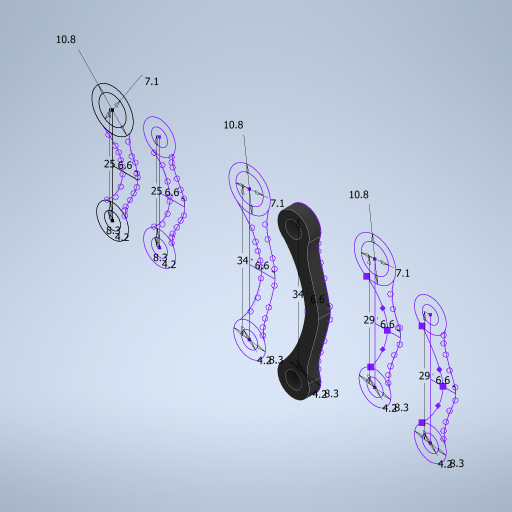
# Autodesk Inventor part: Leg_Front_V5_b
Saved by Autodesk Inventor 2023.1 (Build 271208000, 208)
## iProperties
Created: 2022-10-11
Part Number: Leg_Front_V5_b
Material: Rubber, Silicone
Document SubType Name: Modeling
Designer: Windows10
Density: 1.25 g/cm^3
Appearance: Rubber - Black
Author: Windows10
Autodesk Inventor part; units mm, degrees
ref_plane "YZ Plane" through (0, 0, 0) normal (1, 0, 0) x (0, 1, 0)
ref_plane "XZ Plane" through (0, 0, 0) normal (0, 1, 0) x (-1, 0, 0)
ref_plane "XY Plane" through (0, 0, 0) normal (0, 0, 1) x (1, 0, 0)
sketch "Sketch1" plane through (0, 0, 0) normal (0, 0, 1) x (1, 0, 0)
  circle A0 centre (0, 0) radius 5.4
  line L0 (0, 0) -> (0, -25)
  circle A1 centre (0, -25) radius 4.15
  circle A2 centre (0, -25) radius 2.1
  line L1 (0, -12.5) -> (6.6, -12.5)
  circle A3 centre (0, 0) radius 3.55
  line L2 (4.5636, -2.8868) -> (4.15, -5.0505) construction
  line L3 (4.15, -5.0505) -> (5.1368, -7.8346) construction
  line L4 (5.1368, -7.8346) -> (6.0268, -8.8456) construction
  line L5 (6.0268, -8.8456) -> (6.4445, -11.0297) construction
  line L6 (6.4445, -11.0297) -> (6.6598, -11.8582) construction
  line L7 (6.6598, -11.8582) -> (6.6, -12.5) construction
  spline S0 degree 4 poles (4.5636, -2.8868) (4.15, -5.0505) (5.1368, -7.8346) (6.0268, -8.8456) (6.4445, -11.0297) (6.6598, -11.8582) (6.6, -12.5) knots 1 1 1 1 1 2 3 4 4 4 4 4
  line L8 (-2.6712, -4.6931) -> (-0.9445, -6.0036) construction
  line L9 (-0.9445, -6.0036) -> (0.8697, -7.604) construction
  line L10 (0.8697, -7.604) -> (1.7388, -8.6572) construction
  line L11 (1.7388, -8.6572) -> (2.2595, -10.1019) construction
  line L12 (2.2595, -10.1019) -> (2.7672, -11.4262) construction
  line L13 (2.7672, -11.4262) -> (2.7672, -12.5) construction
  spline S1 degree 4 poles (-2.6712, -4.6931) (-0.9445, -6.0036) (0.8697, -7.604) (1.7388, -8.6572) (2.2595, -10.1019) (2.7672, -11.4262) (2.7672, -12.5) knots 1 1 1 1 1 2 3 4 4 4 4 4
  line L14 (2.7672, -12.5) -> (2.7672, -13.0618) construction
  line L15 (2.7672, -13.0618) -> (2.2595, -16.1544) construction
  line L16 (2.2595, -16.1544) -> (0.8697, -19.1754) construction
  line L17 (0.8697, -19.1754) -> (-1.323, -20.85) construction
  line L18 (-1.323, -20.85) -> (-2.1, -21.4205) construction
  spline S2 degree 4 poles (2.7672, -12.5) (2.7672, -13.0618) (2.2595, -16.1544) (0.8697, -19.1754) (-1.323, -20.85) (-2.1, -21.4205) knots 1 1 1 1 1 2 3 3 3 3 3
  line L19 (6.6, -12.5) -> (6.4445, -14.1704) construction
  line L20 (6.4445, -14.1704) -> (5.6131, -15.9877) construction
  line L21 (5.6131, -15.9877) -> (4.6434, -17.9759) construction
  line L22 (4.6434, -17.9759) -> (3.55, -20.0127) construction
  line L23 (3.55, -20.0127) -> (3.3, -20.9586) construction
  line L24 (3.3, -20.9586) -> (3.3, -22.207) construction
  line L25 (3.3, -22.207) -> (3.7922, -23.3143) construction
  spline S3 degree 4 poles (6.6, -12.5) (6.4445, -14.1704) (5.6131, -15.9877) (4.6434, -17.9759) (3.55, -20.0127) (3.3, -20.9586) (3.3, -22.207) (3.7922, -23.3143) knots 1 1 1 1 1 2 3 4 5 5 5 5 5
  circle A4 centre (35.7502, 0) radius 5.4
  circle A5 centre (35.7502, 0) radius 3.55
  line L26 (12.2485, 0) -> (12.2485, -25)
  circle A6 centre (12.2485, -25) radius 4.15
  circle A7 centre (12.2485, -25) radius 2.1
  line L27 (12.2485, -12.5) -> (18.8485, -12.5)
  line L28 (15.0157, -12.5) -> (15.0157, -13.0618) construction
  line L29 (15.0157, -13.0618) -> (14.5079, -16.1544) construction
  line L30 (14.5079, -16.1544) -> (13.1182, -19.1754) construction
  line L31 (13.1182, -19.1754) -> (10.9255, -20.85) construction
  line L32 (10.9255, -20.85) -> (10.1485, -21.4205) construction
  spline S4 degree 4 poles (15.0157, -12.5) (15.0157, -13.0618) (14.5079, -16.1544) (13.1182, -19.1754) (10.9255, -20.85) (10.1485, -21.4205) knots 1 1 1 1 1 2 3 3 3 3 3
  line L33 (18.8485, -12.5) -> (18.7327, -14.3682) construction
  line L34 (18.7327, -14.3682) -> (17.8616, -15.9877) construction
  line L35 (17.8616, -15.9877) -> (16.8918, -17.9759) construction
  line L36 (16.8918, -17.9759) -> (15.7985, -20.0127) construction
  line L37 (15.7985, -20.0127) -> (15.5485, -20.9586) construction
  line L38 (15.5485, -20.9586) -> (15.5485, -22.207) construction
  line L39 (15.5485, -22.207) -> (16.0407, -23.3143) construction
  spline S5 degree 4 poles (18.8485, -12.5) (18.7327, -14.3682) (17.8616, -15.9877) (16.8918, -17.9759) (15.7985, -20.0127) (15.5485, -20.9586) (15.5485, -22.207) (16.0407, -23.3143) knots 1 1 1 1 1 2 3 4 5 5 5 5 5
  line L40 (18.8485, -12.5) -> (18.7327, -10.6318) construction
  spline S6 degree 4 poles (18.8485, -12.5) (18.7327, -10.6318) (17.8616, -9.0123) (16.8918, -7.0241) (15.7985, -4.9873) (15.5485, -4.0414) (15.5485, -2.793) (16.0407, -1.6857) knots 1 1 1 1 1 2 3 4 5 5 5 5 5
  line L41 (18.7327, -10.6318) -> (17.8616, -9.0123) construction
  line L42 (17.8616, -9.0123) -> (16.8918, -7.0241) construction
  line L43 (16.8918, -7.0241) -> (15.7985, -4.9873) construction
  line L44 (15.7985, -4.9873) -> (15.5485, -4.0414) construction
  line L45 (15.5485, -4.0414) -> (15.5485, -2.793) construction
  line L46 (15.5485, -2.793) -> (16.0407, -1.6857) construction
  line L47 (14.5079, -8.8456) -> (13.1182, -5.8246) construction
  spline S7 degree 4 poles (15.0157, -12.5) (15.0157, -11.9382) (14.5079, -8.8456) (13.1182, -5.8246) (10.9255, -4.15) (10.1485, -3.5795) knots 1 1 1 1 1 2 3 3 3 3 3
  line L48 (15.0157, -12.5) -> (15.0157, -11.9382) construction
  line L49 (15.0157, -11.9382) -> (14.5079, -8.8456) construction
  line L50 (13.1182, -5.8246) -> (10.9255, -4.15) construction
  line L51 (10.9255, -4.15) -> (10.1485, -3.5795) construction
  circle A8 centre (12.2485, 0) radius 2.1
  circle A9 centre (12.2485, 0) radius 4.15
  line L52 (35.7502, 0) -> (35.7502, -34)
  circle A10 centre (35.7502, -34) radius 2.1
  circle A11 centre (35.7502, -34) radius 4.15
  line L53 (35.7502, -17) -> (42.3502, -17)
  line L54 (40.7252, -2.1) -> (39.9002, -5.8246) construction
  line L55 (39.9002, -5.8246) -> (40.5798, -8.8456) construction
  line L56 (40.5798, -8.8456) -> (41.8697, -12.5) construction
  line L57 (41.8697, -12.5) -> (42.3502, -14.707) construction
  line L58 (42.3502, -14.707) -> (42.3502, -17) construction
  spline S8 degree 4 poles (40.7252, -2.1) (39.9002, -5.8246) (40.5798, -8.8456) (41.8697, -12.5) (42.3502, -14.707) (42.3502, -17) knots 1 1 1 1 1 2 3 3 3 3 3
  line L59 (32.2762, -4.1341) -> (36.4644, -8.3401) construction
  line L60 (36.4644, -8.3401) -> (37.406, -11.0297) construction
  line L61 (37.406, -11.0297) -> (38.0185, -12.7794) construction
  line L62 (38.0185, -12.7794) -> (38.6784, -14.6643) construction
  line L63 (38.6784, -14.6643) -> (38.8308, -15.9862) construction
  line L64 (38.8308, -15.9862) -> (38.8308, -17) construction
  spline S9 degree 4 poles (32.2762, -4.1341) (36.4644, -8.3401) (37.406, -11.0297) (38.0185, -12.7794) (38.6784, -14.6643) (38.8308, -15.9862) (38.8308, -17) knots 1 1 1 1 1 2 3 4 4 4 4 4
  line L65 (38.8308, -17) -> (38.8308, -18.5598) construction
  line L66 (38.8308, -18.5598) -> (38.0185, -23.3143) construction
  line L67 (38.0185, -23.3143) -> (36.1571, -27.3727) construction
  line L68 (36.1571, -27.3727) -> (33.2415, -30.6942) construction
  spline S10 degree 4 poles (38.8308, -17) (38.8308, -18.5598) (38.0185, -23.3143) (36.1571, -27.3727) (33.2415, -30.6942) knots 1 1 1 1 1 2 2 2 2 2
  line L69 (42.3502, -17) -> (42.3502, -18.4687) construction
  line L70 (42.3502, -18.4687) -> (40.8654, -24.0864) construction
  line L71 (40.8654, -24.0864) -> (39.9002, -27.1) construction
  line L72 (39.9002, -27.1) -> (39.3002, -29.3894) construction
  line L73 (39.3002, -29.3894) -> (39.3002, -31.2196) construction
  line L74 (39.3002, -31.2196) -> (39.758, -32.9229) construction
  spline S11 degree 4 poles (42.3502, -17) (42.3502, -18.4687) (40.8654, -24.0864) (39.9002, -27.1) (39.3002, -29.3894) (39.3002, -31.2196) (39.758, -32.9229) knots 1 1 1 1 1 2 3 4 4 4 4 4
  line L75 (50.1975, -0.3995) -> (50.1975, -34.3995)
  circle A12 centre (50.1975, -34.3995) radius 2.1
  circle A13 centre (50.1975, -34.3995) radius 4.15
  line L76 (50.1975, -17.3995) -> (56.7975, -17.3995)
  line L77 (53.2781, -17.3995) -> (53.2781, -18.9593) construction
  line L78 (53.2781, -18.9593) -> (52.4658, -23.7138) construction
  line L79 (52.4658, -23.7138) -> (50.6044, -27.7721) construction
  line L80 (50.6044, -27.7721) -> (47.6887, -31.0936) construction
  spline S12 degree 4 poles (53.2781, -17.3995) (53.2781, -18.9593) (52.4658, -23.7138) (50.6044, -27.7721) (47.6887, -31.0936) knots 1 1 1 1 1 2 2 2 2 2
  line L81 (56.7975, -17.3995) -> (56.7975, -18.8682) construction
  line L82 (56.7975, -18.8682) -> (55.3127, -24.4859) construction
  line L83 (55.3127, -24.4859) -> (54.3475, -27.4995) construction
  line L84 (54.3475, -27.4995) -> (53.7475, -29.7889) construction
  line L85 (53.7475, -29.7889) -> (53.7475, -31.619) construction
  line L86 (53.7475, -31.619) -> (54.2053, -33.3224) construction
  spline S13 degree 4 poles (56.7975, -17.3995) (56.7975, -18.8682) (55.3127, -24.4859) (54.3475, -27.4995) (53.7475, -29.7889) (53.7475, -31.619) (54.2053, -33.3224) knots 1 1 1 1 1 2 3 4 4 4 4 4
  line L87 (56.7975, -17.3995) -> (56.7975, -15.9308) construction
  spline S14 degree 4 poles (56.7975, -17.3995) (56.7975, -15.9308) (55.3127, -10.3131) (54.3475, -7.2995) (53.7475, -5.0101) (53.7475, -3.1799) (54.2053, -1.4766) knots 1 1 1 1 1 2 3 4 4 4 4 4
  line L88 (56.7975, -15.9308) -> (55.3127, -10.3131) construction
  line L89 (55.3127, -10.3131) -> (54.3475, -7.2995) construction
  line L90 (54.3475, -7.2995) -> (53.7475, -5.0101) construction
  line L91 (53.7475, -5.0101) -> (53.7475, -3.1799) construction
  line L92 (53.7475, -3.1799) -> (54.2053, -1.4766) construction
  line L93 (53.2781, -17.3995) -> (53.2781, -15.8397) construction
  spline S15 degree 4 poles (53.2781, -17.3995) (53.2781, -15.8397) (52.4658, -11.0852) (50.6044, -7.0268) (47.6887, -3.7053) knots 1 1 1 1 1 2 2 2 2 2
  line L94 (53.2781, -15.8397) -> (52.4658, -11.0852) construction
  line L95 (52.4658, -11.0852) -> (50.6044, -7.0268) construction
  line L96 (50.6044, -7.0268) -> (47.6887, -3.7053) construction
  circle A14 centre (50.1975, -0.3995) radius 2.1
  circle A15 centre (50.1975, -0.3995) radius 4.15
  circle A16 centre (68.4548, 0.5836) radius 5.4
  circle A17 centre (68.4548, 0.5836) radius 3.55
  line L97 (68.4548, 0.5836) -> (68.4548, -28.4164)
  circle A18 centre (68.4548, -28.4164) radius 2.1
  circle A19 centre (68.4548, -28.4164) radius 4.15
  line L98 (68.4548, -13.9164) -> (75.0548, -13.9164)
  line L99 (73.4297, -1.5164) -> (72.6048, -5.241) construction
  line L100 (72.6048, -5.241) -> (73.2844, -8.262) construction
  line L101 (73.2844, -8.262) -> (74.5743, -11.9164) construction
  line L102 (74.5743, -11.9164) -> (75.0548, -11.6234) construction
  line L103 (75.0548, -11.6234) -> (75.0548, -13.9164) construction
  spline S16 degree 4 poles (73.4297, -1.5164) (72.6048, -5.241) (73.2844, -8.262) (74.5743, -11.9164) (75.0548, -11.6234) (75.0548, -13.9164) knots 1 1 1 1 1 2 3 3 3 3 3
  line L104 (75.0548, -13.9164) -> (75.0548, -15.3851) construction
  line L105 (75.0548, -15.3851) -> (73.57, -18.5028) construction
  line L106 (73.57, -18.5028) -> (72.6048, -21.5164) construction
  line L107 (72.6048, -21.5164) -> (72.0048, -23.8058) construction
  line L108 (72.0048, -23.8058) -> (72.0048, -25.636) construction
  line L109 (72.0048, -25.636) -> (72.4626, -27.3393) construction
  spline S17 degree 4 poles (75.0548, -13.9164) (75.0548, -15.3851) (73.57, -18.5028) (72.6048, -21.5164) (72.0048, -23.8058) (72.0048, -25.636) (72.4626, -27.3393) knots 1 1 1 1 1 2 3 4 4 4 4 4
  line L110 (89.5021, -19.3159) -> (89.5021, -20.7846) construction
  spline S18 degree 4 poles (89.5021, -19.3159) (89.5021, -20.7846) (88.0172, -23.9023) (87.0521, -26.9159) (86.4521, -29.2053) (86.4521, -31.0355) (86.9099, -32.7388) knots 1 1 1 1 1 2 3 4 4 4 4 4
  line L111 (89.5021, -20.7846) -> (88.0172, -23.9023) construction
  line L112 (88.0172, -23.9023) -> (87.0521, -26.9159) construction
  line L113 (87.0521, -26.9159) -> (86.4521, -29.2053) construction
  line L114 (86.4521, -29.2053) -> (86.4521, -31.0355) construction
  line L115 (86.4521, -31.0355) -> (86.9099, -32.7388) construction
  line L116 (82.9021, -19.3159) -> (89.5021, -19.3159)
  line L117 (82.9021, -4.8159) -> (82.9021, -33.8159)
  circle A20 centre (82.9021, -33.8159) radius 2.1
  circle A21 centre (82.9021, -33.8159) radius 4.15
  spline S19 degree 4 poles (89.5021, -19.3159) (89.5021, -17.8472) (88.0172, -14.7295) (87.0521, -11.7159) (86.4521, -9.4265) (86.4521, -7.5964) (86.9099, -5.893) knots 1 1 1 1 1 2 3 4 4 4 4 4
  line L118 (89.5021, -19.3159) -> (89.5021, -17.8472) construction
  line L119 (89.5021, -17.8472) -> (88.0172, -14.7295) construction
  line L120 (88.0172, -14.7295) -> (87.0521, -11.7159) construction
  line L121 (87.0521, -11.7159) -> (86.4521, -9.4265) construction
  line L122 (86.4521, -9.4265) -> (86.4521, -7.5964) construction
  line L123 (86.4521, -7.5964) -> (86.9099, -5.893) construction
  circle A22 centre (82.9021, -4.8159) radius 4.15
  circle A23 centre (82.9021, -4.8159) radius 2.1
  spline S20 degree 2 poles (80.8021, -8.3954) (86.1209, -15.5699) (86.2021, -19.3159) knots 0 0 0 1 1 1
  spline S21 degree 2 poles (80.8021, -30.2365) (86.0382, -24.7359) (86.2021, -19.3159) knots 0 0 0 1 1 1
  spline S22 degree 2 poles (67.394, -24.4043) (71.2801, -19.0052) (71.7548, -13.9164) knots 0 0 0 1 1 1
  spline S23 degree 2 poles (66.3548, -4.3914) (71.6414, -8.8733) (71.7548, -13.9164) knots 0 0 0 1 1 1
  point P0 (53.2056, -19.8995)
  point P1 (85.3498, -15.891)
  point P2 (85.0021, -24.2664)
  point P3 (70.5719, -18.7259)
  point P4 (70.5719, -9.4265)
  dimension "d0" = 10.8
  dimension "d1" = 25
  dimension "d2" = 8.3
  dimension "d3" = 4.2
  dimension "d4" = 6.6
  dimension "d5" = 7.1
  dimension "d8" = 10.8
  dimension "d9" = 7.1
  dimension "d11" = 25
  dimension "d12" = 8.3
  dimension "d13" = 4.2
  dimension "d14" = 6.6
  dimension "d18" = 34
  dimension "d19" = 4.2
  dimension "d20" = 8.3
  dimension "d21" = 6.6
  dimension "d24" = 34
  dimension "d25" = 4.2
  dimension "d26" = 8.3
  dimension "d27" = 6.6
  dimension "d32" = 10.8
  dimension "d33" = 7.1
  dimension "d34" = 29
  dimension "d35" = 4.2
  dimension "d36" = 8.3
  dimension "d37" = 6.6
  dimension "d38" = 29
  dimension "d39" = 4.2
  dimension "d40" = 8.3
  dimension "d41" = 6.6
  constraints: 34 symmetric about line, 24 centre point, 24 end point, 24 point on circle, 22 vertical, 19 coincident, 8 midpoint, 6 horizontal, 6 tangent, 4 point on line, 2 perpendicular, 1 collinear, 78 other
  measures "d0" diameter of A0
  measures "d1" distance of L0.start L0.end
  measures "d2" diameter of A1
  measures "d3" diameter of A2
  measures "d4" distance of L1.start L1.end
  measures "d5" diameter of A3
  measures "d8" diameter of A4
  measures "d9" diameter of A5
  measures "d11" distance of L26.start L26.end
  measures "d12" diameter of A6
  measures "d13" diameter of A7
  measures "d14" distance of L27.start L33.start
  measures "d18" distance of L52.start L52.end
  measures "d19" diameter of A10
  measures "d20" diameter of A11
  measures "d21" distance of L53.start L53.end
  measures "d24" distance of L75.start L75.end
  measures "d25" diameter of A12
  measures "d26" diameter of A13
  measures "d27" distance of L76.start L81.start
  measures "d32" diameter of A16
  measures "d33" diameter of A17
  measures "d34" distance of L97.start L97.end
  measures "d35" diameter of A18
  measures "d36" diameter of A19
  measures "d37" distance of L98.start L98.end
  measures "d38" distance of L117.start L117.end
  measures "d39" diameter of A20
  measures "d40" diameter of A21
  measures "d41" distance of L116.start L110.start
extrude "Extrusion1" add sketch "Sketch1" along normal blind 3 contours A0 | A0 L0 S1 | S0 L1 S1 L0 A0 | S3 A1 L0 S2 L1 | A1 | L0 A1 S2
extrude "Extrusion2" add sketch "Sketch1" along normal blind 3 separate body contours A9 | A9 S6 L27 S7 L26 | L26 S7 A9 | L27 S5 A6 L26 S4 | L26 A6 S4 | A6
extrude "Extrusion3" add sketch "Sketch1" along normal blind 3 separate body contours A4 | A4 L52 S9 | S8 L53 S9 L52 A4 | S11 A11 L52 S10 L53 | A11 | L52 A11 S10
extrude "Extrusion4" add sketch "Sketch1" along normal blind 3 separate body contours A15 | A15 S14 L76 S15 L75 | L75 S15 A15 | L76 S13 A13 L75 S12 | L75 A13 S12 | A13
extrude "Extrusion5" add sketch "Sketch1" along normal blind 3 separate body contours S18 A21 L117 S21 L116 | L116 S20 L117 A22 S19 | A21 | A22 | A21 S21 L117 | S20 A22 L117
